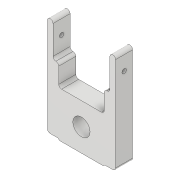
# Autodesk Inventor part: Needle Bearing Mount
Saved by Autodesk Inventor 2018.3 (Build 223284000, 284)
## iProperties
Created: 2018-12-21
Part Number: Needle Bearing Mount
Material: ABS Plastic
Document SubType Name: Modeling
Designer: aye06091
Mass: 93.0627 g
Surface Area: 197.164 cm^2
Volume: 87.795 cm^3
Density: 1.06 g/cm^3
Appearance: Smooth - White
Author: aye06091
Autodesk Inventor part; units mm, degrees
ref_plane "YZ Plane" through (0, 0, 0) normal (1, 0, 0) x (0, 1, 0)
ref_plane "XZ Plane" through (0, 0, 0) normal (0, 1, 0) x (-1, 0, 0)
ref_plane "XY Plane" through (0, 0, 0) normal (0, 0, 1) x (1, 0, 0)
sketch "Sketch1" plane through (0, 0, 0) normal (0, 0, 1) x (1, 0, 0)
  line L0 (0, 0) -> (50.8, 0)
  line L1 (50.8, 0) -> (50.8, -50.8)
  line L2 (50.8, -50.8) -> (0, -50.8)
  line L3 (0, -50.8) -> (0, 0)
  circle A0 centre (25.4, -25.4) radius 9.5885
  dimension "d0" = 19.177
  dimension "d1" = 50.8
  dimension "d2" = 50.8
  dimension "d36" = 25.4
  dimension "d37" = 25.4
  constraints: 8 end point, 2 parallel, 1 centre point, 1 horizontal, 1 perpendicular
  measures "d0" diameter of A0
  measures "d1" distance of L0.end L1.end
  measures "d2" distance of L1.end L2.end
  measures "d36" distance from line of A0.centre L3
  measures "d37" distance from line of A0.centre L2
extrude "Extrusion1" add sketch "Sketch1" against normal blind 19.05
fillet "Fillet1" radius 1.5875 4 edges at (50.8, 0, -9.525) (50.8, -50.8, -9.525) (0, 0, -9.525) (0, -50.8, -9.525)
sketch "Sketch2" plane through (0, -49.2125, 0) normal (-1, 0, 0) x (0, 0, 1)
  line L0 (-19.05, 47.625) -> (0, 47.625)
  line L1 (0, 47.625) -> (0, 0)
  line L2 (0, 0) -> (-19.05, 0)
  line L3 (-19.05, 0) -> (-19.05, 47.625)
  point P0 (0, 49.2125)
  constraints: 8 end point, 2 parallel, 1 horizontal, 1 perpendicular
extrude "Extrusion2" add sketch "Sketch2" along normal blind 12.7
sketch "Sketch3" plane through (-12.7, -1.5875, -19.05) normal (0, 1, 0) x (1, 0, 0)
  line L0 (12.7, 0) -> (0, 0)
  line L1 (0, 0) -> (0, -19.05)
  line L2 (0, -19.05) -> (12.7, -19.05)
  line L3 (12.7, -19.05) -> (12.7, 0)
  constraints: 8 end point, 2 parallel, 1 horizontal, 1 perpendicular
extrude "Extrusion3" add sketch "Sketch3" along normal blind 63.5
sketch "Sketch4" plane through (50.8, -49.2125, 0) normal (1, 0, 0) x (0, 0, -1)
  line L0 (19.05, 0) -> (19.05, -1.5875) projected
  line L1 (0, 47.625) -> (19.05, 47.625)
  line L2 (19.05, 47.625) -> (19.05, 0)
  line L3 (19.05, 0) -> (0, 0)
  line L4 (0, 0) -> (0, 47.625)
  point P0 (0, 49.2125)
  constraints: 8 end point, 2 parallel, 1 horizontal, 1 perpendicular
extrude "Extrusion4" add sketch "Sketch4" along normal blind 12.7
sketch "Sketch5" plane through (50.8, -1.5875, 0) normal (0, 1, 0) x (1, 0, 0)
  line L0 (0, 19.05) -> (12.7, 19.05) projected
  line L1 (12.7, 19.05) -> (0, 19.05)
  line L2 (0, 19.05) -> (0, 0)
  line L3 (0, 0) -> (12.7, 0)
  line L4 (12.7, 0) -> (12.7, 19.05)
  point P0 (-50.8, 0)
  constraints: 8 end point, 2 parallel, 1 horizontal, 1 perpendicular
extrude "Extrusion5" add sketch "Sketch5" along normal blind 63.5
fillet "Fillet3" radius 3.175 1 edges at (50.8, -1.5875, -9.525)
sketch "Sketch7" plane through (-12.7, -49.2125, 0) normal (-1, 0, 0) x (0, 0, 1)
  circle A0 centre (-9.525, 92.075) radius 2.4447
  line L0 (-19.05, 111.125) -> (0, 111.125) projected
  point P0 (0, 49.2125)
  dimension "d20" = 4.8895
  dimension "d38" = 19.05
  constraints: 1 centre point
  measures "d20" diameter of A0
  measures "d38" distance from line of L0 A0.centre
extrude "Extrusion7" cut sketch "Sketch7" against normal blind 101.6
fillet "Fillet7" radius 1.5875 2 edges at (0, -49.2125, -9.525) (50.8, -49.2125, -9.525)
fillet "Fillet9" radius 3.175 2 edges at (-12.7, -49.2125, -9.525) (63.5, -49.2125, -9.525)
sketch "Sketch8" plane through (-12.7, 61.9125, -19.05) normal (0, 1, 0) x (1, 0, 0)
  line L0 (12.7, 0) -> (0, 0) projected
  line L1 (6.35, 0) -> (12.7, 0)
  line L2 (12.7, 0) -> (12.7, -19.05)
  line L3 (12.7, -19.05) -> (6.35, -19.05)
  line L4 (6.35, -19.05) -> (6.35, 0)
  line L5 (63.5, -19.05) -> (76.2, -19.05) projected
  line L6 (63.5, 0) -> (63.5, -19.05) projected
  line L7 (69.85, -19.05) -> (63.5, -19.05)
  line L8 (63.5, -19.05) -> (63.5, 0)
  line L9 (63.5, 0) -> (69.85, 0)
  line L10 (69.85, 0) -> (69.85, -19.05)
  constraints: 16 end point, 4 parallel, 2 horizontal, 2 midpoint, 2 perpendicular
extrude "Extrusion8" cut sketch "Sketch8" against normal blind 38.1
fillet "Fillet10" radius 3.175 4 edges at (-6.35, 23.8125, -9.525) (0, 23.8125, -9.525) (50.8, 23.8125, -9.525) (57.15, 23.8125, -9.525)
fillet "Fillet11" radius 3.175 1 edges at (0, -1.5875, -9.525)
fillet "Fillet12" radius 3.175 4 edges at (63.5, 61.9125, -9.525) (57.15, 61.9125, -9.525) (-6.35, 61.9125, -9.525) (-12.7, 61.9125, -9.525)
body "Solid1"
